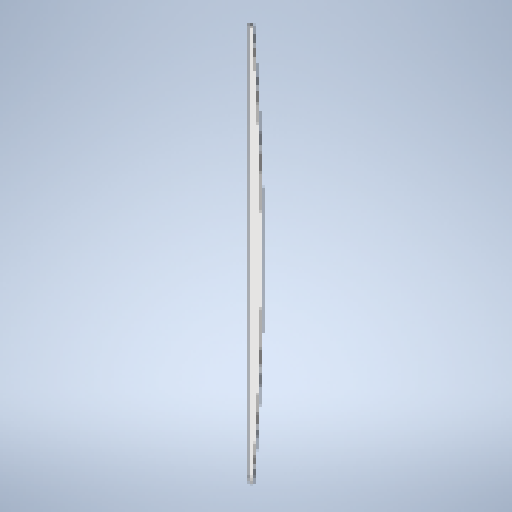
# Autodesk Inventor part: MSC 079 creen pillar
Saved by Autodesk Inventor 2025 (Build 290162010, 162A)
## iProperties
Created: 2024-04-18
Part Number: MSC 079 creen pillar
Material: AISI304
Document SubType Name: Sheet Metal
Designer: admin
Stock Number: МОО 024 лист борт основной
Mass: 48027.3 g
Surface Area: 40202.8 cm^2
Volume: 6003.41 cm^3
Density: 8 g/cm^3
Sheet Metal Rule: AISI304 3mm
Sheet Metal Width: 0,000 mm
Sheet Metal Length: 0,000 mm
Sheet Metal Area: 0,000 mm^2
Appearance: Default
Author: admin
Autodesk Inventor part; units mm, degrees
ref_plane "YZ Plane" through (0, 0, 0) normal (1, 0, 0) x (0, 1, 0)
ref_plane "XZ Plane" through (0, 0, 0) normal (0, 1, 0) x (-1, 0, 0)
ref_plane "XY Plane" through (0, 0, 0) normal (0, 0, 1) x (1, 0, 0)
sketch "Sketch1" plane through (0, 0, 0) normal (0, 0, 1) x (1, 0, 0)
  line L0 (0, 100) -> (0, 50) construction
  line L1 (0, 47) -> (0, 0) construction
  line L2 (0, 50) -> (0, 47) construction
  arc A0 (38, -1950) -> (19, 0) centre (-10977.8747, -1082.2416) ccw
  line L3 (38, -1950) -> (0, -1950)
  line L4 (0, -1950) -> (0, 0)
  line L5 (0, 0) -> (19, 0)
  dimension "d115" = 3
  dimension "d131" = 11050
  dimension "d132" = 19
  dimension "d133" = 38
  dimension "d134" = 1950
  measures "d115" distance of L0.end L1.start
  measures "d131" radius of A0
  measures "d132" distance of L1.end L5.end
  measures "d133" distance of L3.start L3.end
  measures "d134" distance of L1.end L3.end
extrude "Plate3" add sketch "Sketch1" along normal blind 3
sketch "Sketch3" plane through (0, 0, 0) normal (0, 0, -1) x (-1, 0, 0)
  line L0 (0, 0) -> (0, -1950) projected
  line L1 (-19, 0) -> (0, 0) projected
  arc A0 (-19, 0) -> (-38, -1950) centre (10977.8747, -1082.2416) ccw projected
  line L2 (0, -1950) -> (-38, -1950) projected
  circle A1 centre (-8, -1930) radius 3.5
  dimension "d135" = 7
  dimension "d136" = 8
  dimension "d137" = 20
  constraints: 1 centre point
  measures "d135" diameter of A1
  measures "d136" distance from line of L0 A1.centre
  measures "d137" distance from line of L2 A1.centre
extrude "Extrusion2" cut sketch "Sketch3" against normal blind 10 contours A1
pattern_linear "Rectangular Pattern1" count 31 spacing 63 along (0, 1, 0) of "Extrusion2"
equation "\"BendReliefWidth\" = Thickness"
equation "\"BendReliefDepth\" = 0.5 * Thickness"
equation "\"CornerReliefSize\" = 4 * Thickness"
equation "\"MinimumRemnant\" = 2 * Thickness"
equation "\"GapSize\" = Thickness"
equation "\"Thickness\" = 3"
body "Solid4"
